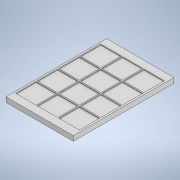
# Autodesk Inventor part: slide substrate rack
Saved by Autodesk Inventor 2020 (Build 240168000, 168)
## iProperties
Created: 2021-07-14
Part Number: slide substrate rack
Material: Generic
Document SubType Name: Modeling
Designer: pab2
Density: 1 g/cm^3
Appearance: Default
Author: pab2
Autodesk Inventor part; units mm, degrees
ref_plane "YZ Plane" through (0, 0, 0) normal (1, 0, 0) x (0, 1, 0)
ref_plane "XZ Plane" through (0, 0, 0) normal (0, 1, 0) x (-1, 0, 0)
ref_plane "XY Plane" through (0, 0, 0) normal (0, 0, 1) x (1, 0, 0)
sketch "Sketch1" plane through (0, 0, 0) normal (0, 1, 0) x (-1, 0, 0)
  line L0 (0, 0) -> (85.48, 0)
  line L1 (85.48, 0) -> (85.48, -127.76)
  line L2 (85.48, -127.76) -> (0, -127.76)
  line L3 (0, -127.76) -> (0, 0)
  line L4 (0, 0) -> (7.0711, -7.0711)
  line L5 (0, 0) -> (10, 0) construction
  circle A0 centre (7.0711, -7.0711) radius 4.7625
  dimension "d0" = 85.48
  dimension "d1" = 127.76
  dimension "offsetDiag" = 10
  dimension "d3" = 45
  dimension "d4" = 9.525
  constraints: 12 end point, 2 horizontal, 2 parallel, 1 centre point, 1 coincident, 1 equal length, 1 perpendicular
  measures "d0" distance of L1.end L2.end
  measures "d1" distance of L0.end L1.end
  measures "offsetDiag" distance of L0.start L4.end
  measures "d3" angle of L4 L5
  measures "d4" diameter of A0
extrude "Extrusion1" add sketch "Sketch1" along normal blind 6.35 contours L0 L1 L2 L3 | A0
sketch "Sketch3" plane through (0, 6.35, 0) normal (0, 1, 0) x (1, 0, 0)
  line L0 (0, 0) -> (0, 127.76) projected
  line L1 (0, 0) -> (-2.3876, 0)
  line L2 (-2.3876, 0) -> (-2.3876, 9.8298)
  line L3 (-2.3876, 9.8298) -> (0, 9.8298)
  line L4 (0, 9.8298) -> (0, 0)
  line L5 (-2.3876, 9.8298) -> (-28.2876, 9.8298)
  line L6 (-28.2876, 9.8298) -> (-28.2876, 35.7298)
  line L7 (-28.2876, 35.7298) -> (-2.3876, 35.7298)
  line L8 (-2.3876, 35.7298) -> (-2.3876, 9.8298)
  line L9 (-28.2876, 35.7298) -> (-29.2876, 35.7298)
  line L10 (-29.2876, 35.7298) -> (-29.2876, 36.7298)
  line L11 (-29.2876, 36.7298) -> (-28.2876, 36.7298)
  line L12 (-28.2876, 36.7298) -> (-28.2876, 35.7298)
  dimension "d23" = 2.3876
  dimension "d24" = 9.8298
  dimension "d25" = 25.9
  dimension "d26" = 25.9
  dimension "d27" = 1
  dimension "d28" = 1
  constraints: 24 end point, 6 parallel, 3 horizontal, 3 perpendicular
  measures "d23" distance of L2.end L3.end
  measures "d24" distance of L1.end L2.end
  measures "d25" distance of L6.end L7.end
  measures "d26" distance of L5.end L6.end
  measures "d27" distance of L10.end L11.end
  measures "d28" distance of L9.end L10.end
extrude "Extrusion2" cut sketch "Sketch3" against normal blind 1 contours L5 L6 L7 L8
pattern_linear "Rectangular Pattern2" count 3 spacing 27.4 along (-1, 0, 0) count 4 spacing 27.4 along (0, 0, -1) of "Extrusion2"
body "Solid1"
